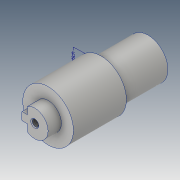
# Autodesk Inventor part: 200-20-ROCKER-CONNECTOR-01
Saved by Autodesk Inventor 2018.2 (Build 222227000, 227)
## iProperties
Manager: feesmrt
Company: FRANC0R
Created: 2017-10-30
Part Number: 200-20-ROCKER-CONNECTOR-01
Material: Aluminium 6061
Document SubType Name: Modeling
Designer: feesmrt
Density: 2.7 g/cm^3
Appearance: Aluminium - flach
Project: Rescue Robot
Cost Center: -
Description: Rocker Profile Connector
Engineer: feesmrt
Authority: feesmrt
Stock Number: 200-20-ROCKER-CONNECTOR-01
Author: feesmrt
Title: Rocker Profile Connector
Subject: Rescue Robot
Revision Number: 1
Autodesk Inventor part; units mm, degrees
ref_plane "YZ Plane" through (0, 0, 0) normal (1, 0, 0) x (0, 1, 0)
ref_plane "XZ Plane" through (0, 0, 0) normal (0, 1, 0) x (-1, 0, 0)
ref_plane "XY Plane" through (0, 0, 0) normal (0, 0, 1) x (1, 0, 0)
derived "200-10-ROCKER-BEARING-01.ipt"
sketch "Skizze_Lagersitz" plane through (0, 0, 0) normal (1, 0, 0) x (0, 1, 0)
  line L0 (-12.5, 36) -> (32.5, 36)
  line L1 (-12.5, -36) -> (-12.5, 36)
  line L2 (-17.5, 32.25) -> (-12.5, 32.25)
  line L3 (-17.5, -32.25) -> (-17.5, 32.25)
  line L4 (-32.5, 18) -> (-17.5, 18)
  line L5 (-32.5, -18) -> (-17.5, -18)
  line L6 (-17.5, -32.25) -> (-12.5, -32.25)
  line L7 (-12.5, -36) -> (32.5, -36)
  line L8 (32.5, 36) -> (32.5, -36)
  line L9 (32.5, 50) -> (32.5, -50)
  line L10 (30, -50) -> (30, 0)
  line L11 (-32.5, -18) -> (-32.5, 18)
  line L12 (-32.5, 50) -> (-32.5, -50)
  line L13 (-32.5, -50) -> (-32.5, 50)
  line L14 (-12.5, -36) -> (-12.5, 36)
  point P0 (0, 0)
  point P1 (30, 86)
  point P2 (30, 14)
  point P3 (-30, 32)
  point P4 (-30, 68)
sketch "Skizze4" plane through (0, 0, 0) normal (1, 0, 0) x (0, 1, 0)
  line L0 (-81.26, 0) -> (51.46, 0) projected
  line L1 (-12.5, -36) -> (-12.5, 36) construction
  line L2 (-32.5, -18) -> (-32.5, 18) construction
  line L3 (22.7, 0) -> (22.7, 15)
  line L4 (22.7, 15) -> (-12.5, 15)
  line L5 (17.7, 0) -> (17.7, 36) construction
  line L6 (-12.5, 15) -> (-12.5, 19)
  line L7 (-12.5, 19) -> (-52.3, 19)
  line L8 (-62.3, 0) -> (22.7, 0)
  line L9 (-62.3, 10) -> (-62.3, 0)
  line L10 (-12.5, 36) -> (32.5, 36) construction
  line L11 (-62.3, 10) -> (-52.3, 10)
  line L12 (-52.3, 10) -> (-52.3, 19)
  point P0 (0, 0)
  dimension "d3" = 30.2
  dimension "d4" = 5
  dimension "d5" = 30
  dimension "d6" = 38
  dimension "d7" = 85
  dimension "d80" = 10
  dimension "d81" = 20
  constraints: 18 end point, 6 point on line, 3 horizontal, 2 perpendicular, 2 vertical, 1 collinear
  measures "d3" distance between parallel lines of L5 L1
  measures "d4" distance between parallel lines of L3 L5
  measures "d5" diameter of L4 L0
  measures "d6" diameter of L7 L0
  measures "d7" distance from line of L9.start L3
  measures "d80" distance between parallel lines of L9 L12
  measures "d81" diameter of L11 L0
revolve "Grundkoerper" add sketch "Skizze4" angle 360 about axis through (0, 0, 0) along (0, 1, 0)
sketch "Skizze11" plane through (0, -62.3, 0) normal (0, -1, 0) x (1, 0, 0)
  circle A0 centre (0, 0) radius 10 projected
hole "M6x12" at (0, -62.3, 0) direction (0, 1, 0) diameter 4.917 depth 17.1 tip angle 118 countersink diameter 6 countersink angle 90 thread size "M6x1" class "6H" standard "ISO Metric profile"
sketch "Skizze12" plane through (0, -62.3, 0) normal (0, -1, 0) x (1, 0, 0)
  line L0 (0, 113.2) -> (0, -77.2) construction
  line L1 (-28.9494, 0) -> (26.9916, 0) construction
  line L2 (-5.4, 3) -> (-5.4, -3) construction
  circle A0 centre (0, 0) radius 10 construction
  line L3 (-5.4, 3) -> (-9.5394, 3)
  line L4 (-5.4, 3) -> (-5.4, 8.4167)
  arc A1 (-5.4, 8.4167) -> (-9.5394, 3) centre (0, 0) ccw
  line L5 (-5.4, -3) -> (-9.5394, -3)
  line L6 (-5.4, -3) -> (-5.4, -8.4167)
  arc A2 (-9.5394, -3) -> (-5.4, -8.4167) centre (0, 0) ccw
  dimension "d76" = 5.4
  dimension "d77" = 6
  constraints: 10 end point, 6 point on circle, 3 symmetric about line, 2 centre point, 1 coincident, 1 horizontal, 1 perpendicular, 1 vertical, 1 other
  measures "d76" distance between parallel lines of L0 L2
  measures "d77" distance of L2.start L2.end
extrude "20x20_Profile_Connector_Cut" cut sketch "Skizze12" against normal blind 10
